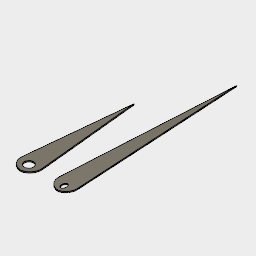
clock hands (Autodesk Fusion 360 design; units mm, degrees)
Autodesk Fusion 360 part; units mm, degrees
note: some values were not read from the file. Chosen so that the rebuilt part matches the saved one: which pieces of a blend or face edit are solid.
sketch "Sketch1" plane through (0, 0, 0) normal (0, 1, 0) x (1, 0, 0)
  line L0 (-50, 50) -> (-55, 0)
  line L1 (-55, 0) -> (-45, 0)
  line L2 (-45, 0) -> (-50, 50)
extrude "Extrude1" add sketch "Sketch1" along normal blind 0.05 makes body 1
extrude "Extrude2" add 1 faces at (-50, 0.05, -16.6667) along direction (0, 1, 0) blind 0.5 on bodies 1 bodies 1
sketch "Sketch2" plane through (0, 0, 0) normal (0, 0, 1) x (1, 0, 0)
fillet "Fillet1" radius 5 4 edges at (-55, 0.275, 0) (-50, 0, 0) (-50, 0.55, 0) (-45, 0.275, 0) on bodies 1
sketch "Sketch3" plane through (0, 0, 0) normal (0, 0, 1) x (1, 0, 0)
sketch "Sketch4" plane through (0, 0.55, 0) normal (0, 1, 0) x (-1, 0, 0)
  arc A0 (49.4751, 0) -> (45.5388, -5.3884) centre (50.514, -4.8909) ccw
  line L0 (45.5388, -5.3884) -> (50, -50)
  line L1 (50, -50) -> (54.4502, -5.4975)
  arc A1 (54.4502, -5.4975) -> (49.4751, 0) centre (49.4751, -5) ccw
  circle A2 centre (50, -4) radius 2
  dimension "d8" = 4
  measures "d8" diameter of A2
extrude "Extrude3" add sketch "Sketch4" along normal blind 1 contours A2 bodies 1
hole "Hole1" at (-50, 1.55, -4) direction (0, -1, 0) diameter 4 depth 8 tip angle 118 bodies 1
sketch "Sketch5" plane through (0, 0, 0) normal (0, 1, 0) x (1, 0, 0)
  line L0 (-40, 0) -> (-31, 0)
  line L1 (-40, 0) -> (-35.5, 78.7064)
  line L2 (-35.5, 78.7064) -> (-31, 0)
extrude "Extrude4" add sketch "Sketch5" along normal blind 0.5 separate body makes body 2
fillet "Fillet2" radius 5 4 edges at (-40, 0.25, 0) (-35.5, 0.5, 0) (-35.5, 0, 0) (-31, 0.25, 0) on bodies 2
sketch "Sketch6" plane through (0, 0.5, 0) normal (0, 1, 0) x (-1, 0, 0)
  arc A0 (34.706, 0) -> (31.2877, -5.0313) centre (36.2795, -4.7459) ccw
  line L0 (31.2877, -5.0313) -> (35.5, -78.7064)
  line L1 (35.5, -78.7064) -> (39.6978, -5.2854)
  arc A1 (39.6978, -5.2854) -> (34.706, 0) centre (34.706, -5) ccw
  ellipse E0 centre (35.2322, -3.0391) end of major axis (35.2322, -1.5391) minor radius 1
  line L2 (35.2322, -4.5391) -> (35.2322, -1.5391)
  line L3 (36.2322, -3.0391) -> (34.2322, -3.0391)
extrude "Extrude5" cut sketch "Sketch6" against normal blind 4.5 contours E0 L2 L3 | E0 L2 L3 | E0 L2 L3 | E0 L2 L3 bodies 2
move_body "Move1" bodies 2 to x (1, 0, 0) y (0, 1, 0) z (0, 0, 1) at (0.9778, 0, -0.5825)
